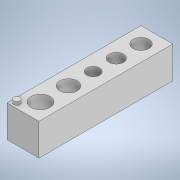
# Autodesk Inventor part: M4 test
Saved by Autodesk Inventor 2021 (Build 250183000, 183)
## iProperties
Created: 2022-11-21
Part Number: M4 test
Material: Generic
Document SubType Name: Modeling
Designer: warre
Density: 1 g/cm^3
Appearance: Default
Author: warre
Autodesk Inventor part; units mm, degrees
ref_plane "YZ Plane" through (0, 0, 0) normal (1, 0, 0) x (0, 1, 0)
ref_plane "XZ Plane" through (0, 0, 0) normal (0, 1, 0) x (-1, 0, 0)
ref_plane "XY Plane" through (0, 0, 0) normal (0, 0, 1) x (1, 0, 0)
sketch "Sketch1" plane through (0, 0, 0) normal (0, 1, 0) x (-1, 0, 0)
  line L0 (5, 22) -> (-5, 22)
  line L1 (-5, 22) -> (-5, -20)
  line L2 (-5, -20) -> (5, -20)
  line L3 (5, -20) -> (5, 22)
  line L4 (0, 0) -> (5, 1) construction
  line L5 (0, 0) -> (-5, 1) construction
  line L6 (0, 0) -> (0, 22) construction
  line L7 (0, 0) -> (0, -20) construction
  dimension "d28" = 5
  dimension "d29" = 5
  dimension "d30" = 20
  dimension "d31" = 22
  constraints: 16 end point, 4 midpoint, 2 parallel, 1 horizontal, 1 perpendicular
  measures "d28" horizontal distance of L4.start L4.end
  measures "d29" horizontal distance of L4.start L5.end
  measures "d30" distance of L4.start L7.end
  measures "d31" distance of L4.start L6.end
extrude "Extrusion1" add sketch "Sketch1" along normal blind 10
sketch "Sketch4" plane through (0, 10, 0) normal (0, 1, 0) x (1, 0, 0)
  circle A0 centre (0, 0) radius 2
  line L0 (0, 2) -> (0, 5) construction
  line L1 (0, 5) -> (0, 7.25) construction
  circle A1 centre (0, 7.25) radius 2.25
  line L2 (0, 9.5) -> (0, 15) construction
  circle A2 centre (0, 15) radius 2.5
  line L3 (0, -2) -> (0, -7.75) construction
  circle A3 centre (0, -7.75) radius 2.75
  line L4 (0, -10.5) -> (0, -16.5) construction
  circle A4 centre (0, -16.5) radius 3
  dimension "d19" = 4.5
  dimension "d23" = 5.5
  dimension "d16" = 4
  dimension "d17" = 3
  dimension "d18" = 2.25
  dimension "d20" = 5.5
  dimension "d21" = 5
  dimension "d22" = 5.75
  dimension "d24" = 6
  dimension "d25" = 6
  constraints: 10 end point, 5 coincident, 5 vertical, 3 centre point, 2 point on circle, 2 vertical alignment, 4 other
  measures "d16" diameter of A0
  measures "d17" distance of L0.start L0.end
  measures "d18" distance of L0.end L1.end
  measures "d20" distance of L2.start L2.end
  measures "d21" diameter of A2
  measures "d22" distance of L3.start L3.end
  measures "d24" distance of L4.start L4.end
  measures "d25" diameter of A4
extrude "Extrusion2" cut sketch "Sketch4" against normal through all
sketch "Sketch6" plane through (0, 10, 0) normal (0, 1, 0) x (1, 0, 0)
  circle A0 centre (-3.5576, -20.41) radius 1
  point P0 (0, 0)
  dimension "d32" = 2
  constraints: 1 centre point
  measures "d32" diameter of A0
extrude "Extrusion3" add sketch "Sketch6" along normal blind 1
body "Solid1"
